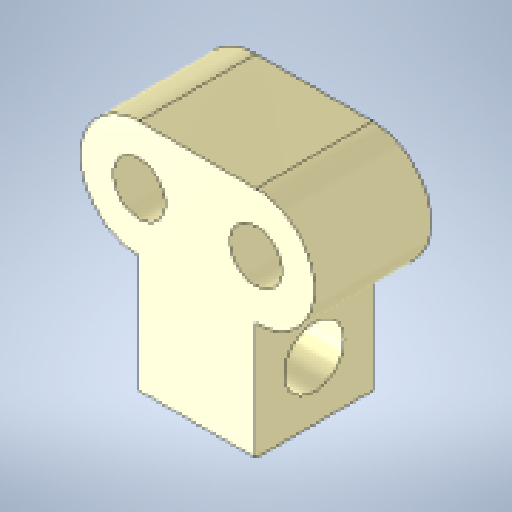
# Autodesk Inventor part: End Guides - Bushing
Saved by Autodesk Inventor 2023.2 (Build 272271000, 271)
## iProperties
Created: 2024-02-24
Part Number: End Guides - Bushing
Material: Nylon 6/6
Document SubType Name: Modeling
Designer: Nathan Cai
Density: 1.13 g/cm^3
Appearance: Nylon 6
Author: Nathan Cai
Autodesk Inventor part; units mm, degrees
ref_plane "YZ Plane" through (0, 0, 0) normal (1, 0, 0) x (0, 1, 0)
ref_plane "XZ Plane" through (0, 0, 0) normal (0, 1, 0) x (-1, 0, 0)
ref_plane "XY Plane" through (0, 0, 0) normal (0, 0, 1) x (1, 0, 0)
sketch "Sketch1" plane through (0, 0, 0) normal (0, 0, 1) x (1, 0, 0)
  line L0 (-3.175, -6.35) -> (3.175, -6.35)
  line L1 (3.175, -6.35) -> (3.175, 6.35)
  line L2 (3.175, 6.35) -> (-3.175, 6.35)
  line L3 (-3.175, 6.35) -> (-3.175, -6.35)
  line L4 (-3.175, -6.35) -> (3.175, 6.35) construction
  line L5 (3.175, -6.35) -> (-3.175, 6.35) construction
  line L6 (-3.175, 3.175) -> (3.175, 3.175) construction
  circle A0 centre (0, 3.175) radius 1.4224
  line L7 (3.175, 6.35) -> (9.525, 6.35)
  line L8 (9.525, 6.35) -> (9.525, 0)
  line L9 (9.525, 0) -> (3.175, 0)
  line L10 (3.175, 0) -> (3.175, 6.35)
  line L11 (9.525, 0) -> (3.175, 6.35) construction
  circle A1 centre (6.35, 3.175) radius 1.4224
  line L12 (0, 0) -> (6.35, 0)
  line L13 (6.35, 0) -> (6.35, -6.35)
  line L14 (6.35, -6.35) -> (0, -6.35)
  line L15 (0, -6.35) -> (0, 0)
  line L16 (0, 0) -> (-3.175, 0)
  arc A2 (-49.8275, -10.2253) -> (-47.6608, -11.7551) centre (-47.0803, -8.6337) ccw projected
  arc A3 (-45.1417, -14.1894) -> (-47.6608, -11.7551) centre (-48.2414, -14.8766) ccw projected
  line L17 (-45.1417, -14.1894) -> (-43.7673, -20.3889) projected
  line L18 (-43.7673, -20.3889) -> (38.3758, -2.1782) projected
  line L19 (38.3758, -2.1782) -> (38.3758, 9.0298) projected
  arc A4 (38.3758, 9.0298) -> (35.9553, 12.1139) centre (35.2008, 9.0298) ccw projected
  line L20 (35.9553, 12.1139) -> (-42.077, 31.2035) projected
  arc A5 (-44.4817, 33.9709) -> (-42.077, 31.2035) centre (-41.3225, 34.2876) ccw projected
  arc A6 (-44.4817, 33.9709) -> (-57.1171, 32.6919) centre (-50.8, 33.3375) ccw projected
  line L21 (-57.1171, 32.6919) -> (-55.856, 20.3523) projected
  arc A7 (-55.856, 20.3523) -> (-54.9425, 18.43) centre (-52.6974, 20.6751) ccw projected
  line L22 (-54.9425, 18.43) -> (-51.7299, 15.2174) projected
  arc A8 (-50.8, 12.9724) -> (-51.7299, 15.2174) centre (-53.975, 12.9724) ccw projected
  line L23 (-50.8, 12.9724) -> (-50.8, -0.2724) projected
  arc A9 (-51.6791, -2.4654) -> (-50.8, -0.2724) centre (-53.975, -0.2724) ccw projected
  arc A10 (-51.6791, -2.4654) -> (-52.1305, -6.2501) centre (-49.3833, -4.6585) ccw projected
  line L24 (-52.1305, -6.2501) -> (-49.8275, -10.2253) projected
  line L25 (22.8045, -0.7521) -> (0.6872, -5.6554) projected
  arc A11 (-3.175, -2.5557) -> (0.6872, -5.6554) centre (0, -2.5557) ccw projected
  line L26 (-3.175, -2.5557) -> (-3.175, -2.3813) projected
  arc A12 (-0.7937, 0) -> (-3.175, -2.3813) centre (-0.7937, -2.3813) ccw projected
  line L27 (-0.7937, 0) -> (6.35, 0) projected
  arc A13 (6.35, 0) -> (6.35, 6.35) centre (6.35, 3.175) ccw projected
  line L28 (6.35, 6.35) -> (-0.7937, 6.35) projected
  arc A14 (-3.175, 8.7312) -> (-0.7937, 6.35) centre (-0.7937, 8.7312) ccw projected
  line L29 (-3.175, 8.7312) -> (-3.175, 12.7383) projected
  arc A15 (0.7545, 15.8224) -> (-3.175, 12.7383) centre (0, 12.7383) ccw projected
  line L30 (0.7545, 15.8224) -> (21.8831, 10.6535) projected
  arc A16 (24.2659, 7.0817) -> (21.8831, 10.6535) centre (21.1286, 7.5695) ccw projected
  arc A17 (24.2659, 7.0817) -> (24.8591, 3.9486) centre (28.9719, 6.35) ccw projected
  arc A18 (22.8045, -0.7521) -> (24.8591, 3.9486) centre (22.1173, 2.3476) ccw projected
  circle A19 centre (28.9719, 6.35) radius 1.4732 projected
  circle A20 centre (-48.0659, -8.3335) radius 1.7526 projected
  circle A21 centre (-33.4336, -15.6589) radius 1.4224 projected
  circle A22 centre (-50.8, 33.3375) radius 3.175 projected
  circle A23 centre (3.7633, -7.4125) radius 1.4224 projected
  circle A24 centre (9.9628, -6.0381) radius 1.4224 projected
  circle A25 centre (16.1622, -4.6637) radius 1.4224 projected
  circle A26 centre (22.3617, -3.2894) radius 1.4224 projected
  line L31 (-15.875, -7.9375) -> (-38.8937, -7.9375) projected
  arc A27 (-42.0687, -4.7625) -> (-38.8937, -7.9375) centre (-38.8937, -4.7625) ccw projected
  line L32 (-42.0687, -4.7625) -> (-42.0687, 17.4625) projected
  arc A28 (-38.8937, 20.6375) -> (-42.0687, 17.4625) centre (-38.8937, 17.4625) ccw projected
  line L33 (-38.8937, 20.6375) -> (-15.875, 20.6375) projected
  arc A29 (-12.7, 17.4625) -> (-15.875, 20.6375) centre (-15.875, 17.4625) ccw projected
  line L34 (-12.7, 17.4625) -> (-12.7, -4.7625) projected
  arc A30 (-15.875, -7.9375) -> (-12.7, -4.7625) centre (-15.875, -4.7625) ccw projected
  circle A31 centre (-7.1437, 17.4625) radius 1.4732 projected
  circle A32 centre (-7.1437, 11.1125) radius 1.4732 projected
  circle A33 centre (-7.1437, 4.7625) radius 1.4732 projected
  circle A34 centre (-7.1437, -1.5875) radius 1.4732 projected
  circle A35 centre (6.35, 3.175) radius 1.4224 projected
  circle A36 centre (0, 3.175) radius 1.4224 projected
  circle A37 centre (3.7633, -7.4125) radius 2.3812
  point P0 (0, -6.35)
  point P1 (1.6322, -6.35)
  point P2 (5.8943, -6.35)
  dimension "d0" = 6.35
  dimension "d1" = 12.7
  dimension "d2" = 3.175
  dimension "d3" = 2.8448
  dimension "d6" = 6.35
  dimension "d7" = 6.35
  dimension "d8" = 2.8448
  constraints: 34 end point, 6 midpoint, 6 parallel, 4 perpendicular, 3 centre point, 3 horizontal, 3 point on line, 1 coincident, 1 tangent
  measures "d0" distance of L2.end L1.end
  measures "d1" distance of L1.end L0.end
  measures "d2" distance between parallel lines of L2 L6
  measures "d3" diameter of A0
  measures "d6" distance of L8.end L9.end
  measures "d7" distance of L7.end L8.end
  measures "d8" diameter of A1
extrude "Extrusion1" add sketch "Sketch1" along normal blind 6.35 contours L15 A11 L25 A37 L0 | A37 L1 A23 L0 | L0 A23 L14 A37 | L15 L12 L1 L25 A11 | A37 L14 A23 L1 | L1 L9 L13 L25 | L25 L13 L14 A37 | L16 L3 L2 L1 L12 | L1 L7 A13 L9 | A13 L8 L9 | L7 L8 A13
fillet "Fillet1" radius 3.175 7 edges at (9.525, 0, 3.175) (9.525, 6.35, 3.175) (-3.175, 6.35, 3.175) (-3.175, 0, 3.175) (5.8943, -6.35, 3.175) (6.35, -6.35, 3.175) (1.6322, -6.35, 3.175)
sketch "Sketch2" plane through (0, -6.35, 0) normal (-1, 0, 0) x (0, 0, 1)
  line L0 (0, 0) -> (0, 6.35) projected
  line L1 (0, 3.175) -> (6.35, 3.175) construction
  line L2 (6.35, 0) -> (6.35, 6.35) projected
  line L3 (0, 0) -> (6.35, 0) projected
  circle A0 centre (3.175, 3.175) radius 1.625
  dimension "d9" = 3.175
  dimension "d10" = 3.25
  constraints: 3 midpoint, 2 end point, 1 centre point, 1 horizontal
  measures "d9" distance between parallel lines of L3 L1
  measures "d10" diameter of A0
extrude "Extrusion2" cut sketch "Sketch2" against normal through all
equation "\"d8\" = d3"
body "Solid1"
